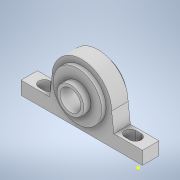
# Autodesk Inventor part: PillowBlockBearing
Saved by Autodesk Inventor 2020 (Build 240168000, 168)
## iProperties
Created: 2020-03-13
Part Number: PillowBlockBearing
Material: Generic
Document SubType Name: Modeling
Designer: jgranlund
Density: 1 g/cm^3
Appearance: Default
Author: jgranlund
Autodesk Inventor part; units mm, degrees
ref_plane "YZ Plane" through (0, 0, 0) normal (1, 0, 0) x (0, 1, 0)
ref_plane "XZ Plane" through (0, 0, 0) normal (0, 1, 0) x (-1, 0, 0)
ref_plane "XY Plane" through (0, 0, 0) normal (0, 0, 1) x (1, 0, 0)
sketch "Sketch1" plane through (0, 0, 0) normal (0, 0, 1) x (1, 0, 0)
  line L0 (-140, 0) -> (-140, 15)
  line L1 (-140, 15) -> (-107, 15)
  line L2 (-33, 15) -> (0, 15)
  line L3 (0, 15) -> (0, 0)
  arc A0 (-35.6047, 36.5) -> (-104.3953, 36.5) centre (-70, 36.5) ccw
  circle A1 centre (-70, 36.5) radius 12.5
  circle A2 centre (-70, 36.5) radius 15.5
  line L4 (-107, 15) -> (-104.3953, 36.5)
  line L5 (-33, 15) -> (-35.6047, 36.5)
  circle A3 centre (-70, 36.5) radius 28
  line L6 (-140, 0) -> (0, 0)
  dimension "d0" = 140
  dimension "d1" = 15
  dimension "d7" = 25
  dimension "d8" = 31
  dimension "d9" = 56
  dimension "d10" = 15
  dimension "d11" = 68.7907
  dimension "d16" = 36.5
  dimension "d17" = 70
  dimension "d20" = 33
  dimension "d21" = 33
  dimension "d22" = 33
  dimension "d23" = 15
  dimension "d24" = 15
  dimension "d26" = 21.5
  dimension "d27" = 21.5
  constraints: 14 end point, 4 centre point, 3 coincident, 2 point on circle, 2 point on line, 1 perpendicular
  measures "d0" distance of L3.end L0.start
  measures "d1" distance of L0.start L0.end
  measures "d7" diameter of A1
  measures "d8" diameter of A2
  measures "d9" diameter of A3
  measures "d10" distance of L2.end L3.end
  measures "d11" diameter of A0
  measures "d16" vertical distance of L3.end A0.centre
  measures "d17" horizontal distance of A0.centre L3.end
  measures "d20" distance of L0.end L1.end
  measures "d21" distance of L2.start L2.end
  measures "d22" horizontal distance of L2.start L3.end
  measures "d23" vertical distance of L3.end L2.start
  measures "d24" vertical distance of L0.start L1.end
  measures "d26" vertical distance of L1.end L4.end
  measures "d27" vertical distance of L2.start L5.end
extrude "Extrusion1" add sketch "Sketch1" along normal mid plane 19 contours L0 L1 L4 A0 L5 L2 L3 L6
sketch "Sketch2" plane through (0, 0, 9.5) normal (0, 0, 1) x (1, 0, 0)
  circle A0 centre (-70, 36.5) radius 15.5
  circle A1 centre (-70, 36.5) radius 28
  point P0 (0, 0)
  dimension "d30" = 36.5
  dimension "d31" = 70
  dimension "d32" = 31
  dimension "d33" = 56
  constraints: 2 centre point, 1 coincident
  measures "d30" vertical distance of point (0, 0) A0.centre
  measures "d31" horizontal distance of A0.centre point (0, 0)
  measures "d32" diameter of A0
  measures "d33" diameter of A1
extrude "Extrusion2" add sketch "Sketch2" along normal blind 5
sketch "Sketch3" plane through (-70, 36.5, 14.5) normal (0, 0, 1) x (1, 0, 0)
  point P0 (70, -36.5)
sketch "Sketch4" plane through (0, 0, -9.5) normal (0, 0, -1) x (-1, 0, 0)
  circle A0 centre (70, 36.5) radius 15.5
  circle A1 centre (70, 36.5) radius 28
  line L0 (140, 0) -> (140, 15) projected
  point P0 (0, 0)
  dimension "d36" = 31
  dimension "d37" = 56
  dimension "d38" = 70
  dimension "d39" = 36.5
  constraints: 2 centre point, 1 coincident
  measures "d36" diameter of A0
  measures "d37" diameter of A1
  measures "d38" distance from line of L0 A0.centre
  measures "d39" vertical distance of L0.start A0.centre
extrude "Extrusion3" add sketch "Sketch4" along normal blind 5
sketch "Sketch5" plane through (0, 0, 0) normal (0, 0, 1) x (1, 0, 0)
  circle A0 centre (-70, 36.5) radius 15.5 projected
  circle A1 centre (-70, 36.5) radius 15.5
  circle A2 centre (-70, 36.5) radius 12.0569
  point P0 (0, 0)
  constraints: 2 centre point, 2 coincident
extrude "Extrusion4" add sketch "Sketch5" along normal mid plane 45
sketch "Sketch6" plane through (-140, 0, 9.5) normal (0, -1, 0) x (1, 0, 0)
  line L0 (0, -19) -> (33, -19) projected
  line L1 (140, -19) -> (140, 0) projected
  line L2 (33, 0) -> (0, 0) projected
  line L3 (140, -19) -> (0, -19) projected
  line L4 (0, -19) -> (0, 0) projected
  arc A0 (17.5, -3) -> (17.5, -16) centre (17.5, -9.5) ccw
  arc A1 (23.5, -16) -> (23.5, -3) centre (23.5, -9.5) ccw
  line L5 (17.5, -3) -> (23.5, -3)
  line L6 (17.5, -16) -> (23.5, -16)
  line L7 (54.5, 0) -> (85.5, 0) projected
  arc A2 (122.5, -16) -> (122.5, -3) centre (122.5, -9.5) ccw
  arc A3 (116.5, -3) -> (116.5, -16) centre (116.5, -9.5) ccw
  line L8 (122.5, -3) -> (116.5, -3)
  line L9 (122.5, -16) -> (116.5, -16)
  point P0 (140, -9.5)
  dimension "d50" = 6.5
  dimension "d51" = 6.5
  dimension "d52" = 6.5
  dimension "d53" = 6.5
  dimension "d54" = 6
  dimension "d55" = 6
  dimension "d56" = 6
  dimension "d57" = 6
  dimension "d58" = 17.5
  dimension "d59" = 17.5
  dimension "d60" = 9.5
  dimension "d61" = 9.5
  dimension "d62" = 17.5
  dimension "d63" = 17.5
  dimension "d64" = 17.5
  dimension "d65" = 3
  dimension "d66" = 3
  dimension "d67" = 6
  constraints: 8 end point, 8 point on circle, 4 centre point, 2 horizontal
  measures "d50" radius of A0
  measures "d51" radius of A2
  measures "d52" radius of A3
  measures "d53" radius of A1
  measures "d54" distance of L5.start L5.end
  measures "d55" distance of L6.start L6.end
  measures "d56" distance of L9.start L9.end
  measures "d57" distance of L8.start L8.end
  measures "d58" horizontal distance of A2.centre L1.end
  measures "d59" horizontal distance of A0.centre L2.end
  measures "d60" vertical distance of A0.centre L2.end
  measures "d61" vertical distance of A2.centre L1.end
  measures "d62" horizontal distance of L1.start L9.start
  measures "d63" horizontal distance of L0.start L6.start
  measures "d64" horizontal distance of L1.end L8.start
  measures "d65" vertical distance of L1.end L8.end
  measures "d66" vertical distance of L2.end L5.start
  measures "d67" distance of A2.centre A3.centre
extrude "Extrusion5" cut sketch "Sketch6" against normal through all
body "Solid1"
